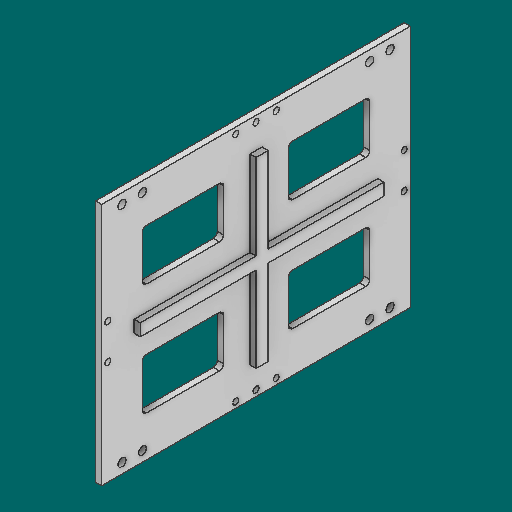
# Autodesk Inventor part: back_plate
Saved by Autodesk Inventor 2026.1 (Build 301233000, 233)
## iProperties
Created: 2025-11-06
Part Number: back_plate
Material: Generic
Document SubType Name: Modeling
Designer: emanuel
Density: 1 g/cm^3
Appearance: Default
Author: emanuel
Autodesk Inventor part; units mm, degrees
ref_plane "YZ Plane" through (0, 0, 0) normal (1, 0, 0) x (0, 1, 0)
ref_plane "XZ Plane" through (0, 0, 0) normal (0, 1, 0) x (-1, 0, 0)
ref_plane "XY Plane" through (0, 0, 0) normal (0, 0, 1) x (1, 0, 0)
sketch "Sketch1" plane through (0, 0, 0) normal (1, 0, 0) x (0, 1, 0)
  line L0 (0, 0) -> (17.4, 0)
  line L1 (17.4, 0) -> (17.4, -146)
  line L2 (17.4, -146) -> (0, -146)
  line L3 (0, -146) -> (0, 0)
  circle A0 centre (17.4, 0) radius 1.5
  circle A1 centre (0, 0) radius 1.5
  circle A2 centre (17.4, -146) radius 1.5
  circle A3 centre (0, -146) radius 1.5
  line L4 (17.4, -146) -> (20.4, -146)
  line L5 (20.4, -146) -> (20.4, -149)
  line L6 (20.4, -149) -> (17.4, -149)
  line L7 (17.4, -149) -> (17.4, -146)
  line L8 (0, 0) -> (-3, 0)
  line L9 (-3, 0) -> (-3, 3)
  line L10 (-3, 3) -> (0, 3)
  line L11 (0, 3) -> (0, 0)
  line L12 (-3, 3) -> (20.4, 3)
  line L13 (20.4, 3) -> (20.4, -149)
  line L14 (20.4, -149) -> (-3, -149)
  line L15 (-3, -149) -> (-3, 3)
  line L16 (20.4, 3) -> (68.7, 3)
  line L17 (68.7, 3) -> (68.7, -149)
  line L18 (68.7, -149) -> (20.4, -149)
  line L19 (20.4, -149) -> (20.4, 3)
  line L20 (-3, -149) -> (-51.3, -149)
  line L21 (-51.3, -149) -> (-51.3, 3)
  line L22 (-51.3, 3) -> (-3, 3)
  line L23 (-3, 3) -> (-3, -149)
  line L24 (68.7, -73) -> (65.7, -73)
  line L25 (65.7, -73) -> (65.7, -63)
  line L26 (65.7, -63) -> (65.7, -83)
  circle A4 centre (65.7, -63) radius 1.5
  circle A5 centre (65.7, -73) radius 1.5
  circle A6 centre (65.7, -83) radius 1.5
  line L27 (65.7, -73) -> (62.7, -73)
  line L28 (-48.3, -73) -> (-48.3, -63)
  line L29 (-48.3, -63) -> (-48.3, -83)
  circle A7 centre (-48.3, -63) radius 1.5
  circle A8 centre (-48.3, -73) radius 1.5
  circle A9 centre (-48.3, -83) radius 1.5
  line L30 (-48.3, -73) -> (-51.3, -73)
  dimension "d0" = 17.4
  dimension "d1" = 146
  dimension "d2" = 3
  dimension "d3" = 3
  dimension "d4" = 3
  dimension "d5" = 3
  dimension "d6" = 3
  dimension "d7" = 3
  dimension "d8" = 3
  dimension "d9" = 3
  dimension "d10" = 48.3
  dimension "d11" = 48.3
  dimension "d12" = 3
  dimension "d13" = 10
  dimension "d14" = 20
  dimension "d15" = 3
  dimension "d16" = 3
  dimension "d17" = 3
  dimension "d18" = 3
  dimension "d19" = 10
  dimension "d20" = 20
  dimension "d21" = 3
  dimension "d22" = 3
  dimension "d23" = 3
  dimension "d24" = 3
  constraints: 62 end point, 12 parallel, 10 centre point, 10 coincident, 9 horizontal, 7 perpendicular, 3 point on line, 1 midpoint
  measures "d0" distance of L1.end L2.end
  measures "d1" distance of L0.end L1.end
  measures "d2" diameter of A0
  measures "d3" diameter of A1
  measures "d4" diameter of A2
  measures "d5" diameter of A3
  measures "d6" distance of L5.end L6.end
  measures "d7" distance of L4.end L5.end
  measures "d8" distance of L9.end L10.end
  measures "d9" distance of L8.end L9.end
  measures "d10" distance of L17.end L18.end
  measures "d11" distance of L21.end L22.end
  measures "d12" distance of L24.start L24.end
  measures "d13" distance of L24.end L25.end
  measures "d14" distance of L25.end L26.end
  measures "d15" diameter of A4
  measures "d16" diameter of A5
  measures "d17" diameter of A6
  measures "d18" distance of L27.start L27.end
  measures "d19" distance of L28.start L29.start
  measures "d20" distance of L29.start L29.end
  measures "d21" diameter of A7
  measures "d22" diameter of A8
  measures "d23" diameter of A9
  measures "d24" distance of L30.start L30.end
extrude "Extrusion1" add sketch "Sketch1" along normal blind 3 contours A1 L11 L12 L13 L4 A2 L1 A0 L0 | L0 A0 L1 A2 L2 A3 L3 A1 | L3 A3 L2 A2 L7 L14 L15 L8 A1 | L8 L9 L10 L11 A1 | L15 L20 L21 L22 L9 | L16 L17 L18 L5 L13 | L7 A2 L4 L5 L6
sketch "Sketch2" plane through (3, 0, 0) normal (1, 0, 0) x (0, 0, -1)
  line L0 (-3, 68.7) -> (-3, -51.3) projected
  line L1 (-3, 8.7) -> (149, 8.7)
  line L2 (149, -51.3) -> (149, 68.7) projected
  line L3 (13, 11.7) -> (133, 11.7)
  line L4 (133, 11.7) -> (133, 5.7)
  line L5 (133, 5.7) -> (13, 5.7)
  line L6 (13, 5.7) -> (13, 11.7)
  line L7 (13, 11.7) -> (133, 5.7) construction
  line L8 (133, 11.7) -> (13, 5.7) construction
  line L9 (70, -36.3) -> (76, -36.3)
  line L10 (76, -36.3) -> (76, 53.7)
  line L11 (76, 53.7) -> (70, 53.7)
  line L12 (70, 53.7) -> (70, -36.3)
  line L13 (70, -36.3) -> (76, 53.7) construction
  line L14 (76, -36.3) -> (70, 53.7) construction
  point P0 (0, 0)
  point P1 (73, 8.7)
  point P2 (73, 8.7)
  point P3 (76, 5.7)
  point P4 (76, 11.7)
  point P5 (70, 11.7)
  point P6 (70, 5.7)
  dimension "d27" = 120
  dimension "d28" = 6
  dimension "d29" = 6
  dimension "d30" = 90
  constraints: 26 end point, 8 midpoint, 4 parallel, 2 horizontal, 2 perpendicular
  measures "d27" distance of L4.end L5.end
  measures "d28" distance of L3.end L4.end
  measures "d29" distance of L11.end L10.end
  measures "d30" distance of L10.end L9.end
extrude "Extrusion2" add sketch "Sketch2" along normal blind 3
sketch "Sketch3" plane through (3, 0, 0) normal (1, 0, 0) x (0, 0, -1)
  line L0 (-3, 68.7) -> (-3, -51.3) projected
  line L1 (-3, 68.7) -> (17, 68.7)
  line L2 (17, 68.7) -> (17, 48.7)
  line L3 (17, 48.7) -> (-3, 48.7)
  line L4 (-3, 48.7) -> (-3, 68.7)
  line L5 (17, 48.7) -> (57, 48.7)
  line L6 (57, 48.7) -> (57, 23.7)
  line L7 (57, 23.7) -> (17, 23.7)
  line L8 (17, 23.7) -> (17, 48.7)
  line L9 (149, -51.3) -> (149, 68.7) projected
  line L10 (149, 68.7) -> (129, 68.7)
  line L11 (129, 68.7) -> (129, 48.7)
  line L12 (129, 48.7) -> (149, 48.7)
  line L13 (149, 48.7) -> (149, 68.7)
  line L14 (129, 48.7) -> (89, 48.7)
  line L15 (89, 48.7) -> (89, 23.7)
  line L16 (89, 23.7) -> (129, 23.7)
  line L17 (129, 23.7) -> (129, 48.7)
  line L18 (-3, -51.3) -> (17, -51.3)
  line L19 (17, -51.3) -> (17, -31.3)
  line L20 (17, -31.3) -> (-3, -31.3)
  line L21 (-3, -31.3) -> (-3, -51.3)
  line L22 (17, -31.3) -> (57, -31.3)
  line L23 (57, -31.3) -> (57, -6.3)
  line L24 (57, -6.3) -> (17, -6.3)
  line L25 (17, -6.3) -> (17, -31.3)
  line L26 (149, -51.3) -> (129, -51.3)
  line L27 (129, -51.3) -> (129, -31.3)
  line L28 (129, -31.3) -> (149, -31.3)
  line L29 (149, -31.3) -> (149, -51.3)
  line L30 (129, -31.3) -> (89, -31.3)
  line L31 (89, -31.3) -> (89, -6.3)
  line L32 (89, -6.3) -> (129, -6.3)
  line L33 (129, -6.3) -> (129, -31.3)
  point P0 (0, 0)
  dimension "d33" = 20
  dimension "d34" = 20
  dimension "d35" = 40
  dimension "d36" = 25
  dimension "d37" = 20
  dimension "d38" = 20
  dimension "d39" = 40
  dimension "d40" = 25
  dimension "d41" = 20
  dimension "d42" = 20
  dimension "d43" = 25
  dimension "d44" = 20
  dimension "d45" = 20
  dimension "d46" = 40
  dimension "d47" = 25
  constraints: 64 end point, 16 parallel, 8 horizontal, 8 perpendicular, 2 point on line
  measures "d33" distance of L2.end L3.end
  measures "d34" distance of L1.end L2.end
  measures "d35" distance of L6.end L7.end
  measures "d36" distance of L5.end L6.end
  measures "d37" distance of L12.end L11.end
  measures "d38" distance of L11.end L10.end
  measures "d39" distance of L16.end L15.end
  measures "d40" distance of L15.end L14.end
  measures "d41" distance of L20.end L19.end
  measures "d42" distance of L19.end L18.end
  measures "d43" distance of L23.end L22.end
  measures "d44" distance of L27.end L28.end
  measures "d45" distance of L26.end L27.end
  measures "d46" distance of L31.end L32.end
  measures "d47" distance of L30.end L31.end
extrude "Extrusion3" cut sketch "Sketch3" against normal blind 3 contours L5 L6 L7 L8 | L25 L24 L23 L22 | L30 L31 L32 L33 | L17 L16 L15 L14
fillet "Fillet1" radius 2 16 edges at (1.5, 23.7, -129) (1.5, 48.7, -129) (1.5, 48.7, -89) (1.5, 23.7, -89) (1.5, 48.7, -57) (1.5, 23.7, -57) (1.5, 48.7, -17) (1.5, 23.7, -17) (1.5, -31.3, -57) (1.5, -6.3, -57) (1.5, -6.3, -17) (1.5, -31.3, -17) (1.5, -31.3, -129) (1.5, -6.3, -129) (1.5, -6.3, -89) (1.5, -31.3, -89)
sketch "Sketch4" plane through (3, 0, 0) normal (1, 0, 0) x (0, 0, -1)
  line L0 (-3, 68.7) -> (-3, -51.3) projected
  line L1 (-3, 68.7) -> (7, 68.7)
  line L2 (7, 68.7) -> (7, 63.7)
  line L3 (7, 63.7) -> (-3, 63.7)
  line L4 (-3, 63.7) -> (-3, 68.7)
  line L5 (149, -51.3) -> (149, 68.7) projected
  line L6 (149, 68.7) -> (139, 68.7)
  line L7 (139, 68.7) -> (139, 63.7)
  line L8 (139, 63.7) -> (149, 63.7)
  line L9 (149, 63.7) -> (149, 68.7)
  line L10 (149, -51.3) -> (139, -51.3)
  line L11 (139, -51.3) -> (139, -46.3)
  line L12 (139, -46.3) -> (149, -46.3)
  line L13 (149, -46.3) -> (149, -51.3)
  line L14 (-3, -51.3) -> (149, -51.3) projected
  line L15 (-3, -51.3) -> (7, -51.3)
  line L16 (7, -51.3) -> (7, -46.3)
  line L17 (7, -46.3) -> (-3, -46.3)
  line L18 (-3, -46.3) -> (-3, -51.3)
  circle A0 centre (7, 63.7) radius 2
  circle A1 centre (139, 63.7) radius 2
  circle A2 centre (139, -46.3) radius 2
  circle A3 centre (7, -46.3) radius 2
  line L19 (7, 63.7) -> (17, 63.7)
  line L20 (139, -46.3) -> (129, -46.3)
  line L21 (17, 63.7) -> (129, 63.7)
  line L22 (129, 63.7) -> (129, -46.3)
  line L23 (129, -46.3) -> (17, -46.3)
  line L24 (17, -46.3) -> (17, 63.7)
  circle A4 centre (129, 63.7) radius 2
  circle A5 centre (17, -46.3) radius 2
  circle A6 centre (17, 63.7) radius 2
  circle A7 centre (129, -46.3) radius 2
  point P0 (0, 0)
  dimension "d51" = 10
  dimension "d52" = 5
  dimension "d53" = 10
  dimension "d54" = 5
  dimension "d55" = 10
  dimension "d56" = 5
  dimension "d57" = 10
  dimension "d58" = 5
  dimension "d59" = 4
  dimension "d60" = 4
  dimension "d61" = 4
  dimension "d62" = 4
  dimension "d63" = 10
  dimension "d64" = 10
  dimension "d65" = 4
  dimension "d66" = 4
  dimension "d67" = 4
  dimension "d68" = 4
  constraints: 44 end point, 10 parallel, 8 centre point, 8 coincident, 7 horizontal, 5 perpendicular
  measures "d51" distance of L2.end L3.end
  measures "d52" distance of L1.end L2.end
  measures "d53" distance of L8.end L7.end
  measures "d54" distance of L7.end L6.end
  measures "d55" distance of L11.end L12.end
  measures "d56" distance of L10.end L11.end
  measures "d57" distance of L17.end L16.end
  measures "d58" distance of L16.end L15.end
  measures "d59" diameter of A0
  measures "d60" diameter of A1
  measures "d61" diameter of A2
  measures "d62" diameter of A3
  measures "d63" distance of L19.start L19.end
  measures "d64" distance of L20.start L20.end
  measures "d65" diameter of A4
  measures "d66" diameter of A5
  measures "d67" diameter of A6
  measures "d68" diameter of A7
extrude "Extrusion4" cut sketch "Sketch4" against normal blind 10 contours A0 L2 L3 | L3 L19 A0 | A0 L19 L2 | A3 L16 L17 | L17 L16 A3 | A6 L21 L19 | L19 L24 A6 | L21 A6 L24 | A2 L20 L11 | L11 L12 A2 | A4 L22 L21 | L21 L22 A4 | A5 L23 L24 | L24 L23 A5 | L20 A2 L12 | A7 L23 L20 | L20 L22 A7 | L22 L23 A7 | A1 L7 L8 | L8 L7 A1
body "Solid1"
